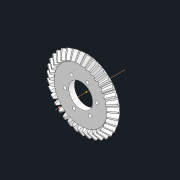
# Autodesk Inventor part: かさ歯車2
Saved by Autodesk Inventor 2021 (Build 250183000, 183)
## iProperties
CustomPartVersion: 1
Created: 2021-07-25
Part Number: かさ歯車2
Material: ABS プラスチック
Document SubType Name: Modeling
Designer: yuto6
Categories: <?xml version="1.0" encoding="UTF-16"?> <MemberInstance><Categories><FamilyTemplate><FamilyTemplateParameter ValueType="xs:double" Id="1" ObjectReferenceKey="da_z" ObjectType="kUserParameterObject"/><FamilyTemplateParameter ValueType="xs:double" Id="2" ObjectReferenceKey="da_b" ObjectType="kUserParameterObject"/><FamilyTemplateParameter ValueType="xs:double" Id="3" ObjectReferenceKey="da_beta" ObjectType="kUserParameterObject"/><FamilyTemplateParameter ValueType="xs:double" Id="4" ObjectReferenceKey="da_dae" ObjectType="kUserParameterObject"/><FamilyTemplateParameter ValueType="xs:double" Id="5" ObjectReferenceKey="da_ve" ObjectType="kUserParameterObject"/><FamilyTemplateParameter ValueType="xs:double" Id="6" ObjectReferenceKey="da_omega" ObjectType="kUserParameterObject"/><FamilyTemplateParameter ValueType="xs:string" Id="7" ObjectReferenceKey="EAIAABAAAAAAHwAAAAAAAIAAAAAAAAAA" ObjectType="83914240" SubObjectId="SurfaceGeometry"/></FamilyTemplate><ParamToTemplateMap><ParamToTemplate CategoryParameter="//CategoryParameter[@InternalName='046C89C9-8512-4d59-83FE-43B91F4F132A']" TemplateParameter="1"/><ParamToTemplate CategoryParameter="//CategoryParameter[@InternalName='2552DF32-E462-4b46-AEBF-C6C7768E72AC']" TemplateParameter="2"/><ParamToTemplate CategoryParameter="//CategoryParameter[@InternalName='C9EE641D-15FC-4fae-A226-E94C4372FDD7']" TemplateParameter="3"/><ParamToTemplate><ParamToTemplate CategoryParameter="//CategoryParameter[@InternalName='00B6519A-459B-49c7-AD84-2E56D39A5744']" ConstantValue="-0.000000"/></ParamToTemplate><ParamToTemplate><ParamToTemplate CategoryParameter="//CategoryParameter[@InternalName='04B31F0E-C7A6-4894-AA32-9629BEFACF47']" ConstantValue="1.000000"/></ParamToTemplate><ParamToTemplate><ParamToTemplate CategoryParameter="//CategoryParameter[@InternalName='43CBEC2E-7847-49e7-A936-2F7889FCB2D9']" ConstantValue="0.200000"/></ParamToTemplate><ParamToTemplate><ParamToTemplate CategoryParameter="//CategoryParameter[@InternalName='B1EFC894-105D-4ebd-86BF-FA20ED196853']" ConstantValue="0.300000"/></ParamToTemplate><ParamToTemplate><ParamToTemplate CategoryParameter="//CategoryParameter[@InternalName='51175063-3D10-4879-93E8-6246FE8B403D']" ConstantValue="2060000000.000000"/></ParamToTemplate><ParamToTemplate><ParamToTemplate CategoryParameter="//CategoryParameter[@InternalName='A3A52E27-4454-46a9-B0BD-C932399B70AF']" ConstantValue="0.300000"/></ParamToTemplate><ParamToTemplate CategoryParameter="//CategoryParameter[@InternalName='2A200944-5A8C-41ca-B96E-8520D2E510F1']" TemplateParameter="4"/><ParamToTemplate><ParamToTemplate CategoryParameter="//CategoryParameter[@InternalName='1A637F62-92C8-44bc-B81F-10802510B579']" ConstantValue="5.719126"/></ParamToTemplate><ParamToTemplate CategoryParameter="//CategoryParameter[@InternalName='B52DD4BE-6863-48fb-BF58-89EF6F9EC65C']" TemplateParameter="5"/><ParamToTemplate><ParamToTemplate CategoryParameter="//CategoryParameter[@InternalName='3956BFF2-84D2-457d-93C2-9B0613DEBA67']" ConstantValue="1.848193"/></ParamToTemplate><ParamToTemplate CategoryParameter="//CategoryParameter[@InternalName='739CFA02-461B-4bf8-8049-181FCAD8B28F']" TemplateParameter="6"/><ParamToTemplate><ParamToTemplate CategoryParameter="//CategoryParameter[@InternalName='A27E999F-E2CE-4481-8A2A-EBF499C4C3C5']" ConstantValue="-0.000000"/></ParamToTemplate><ParamToTemplate><ParamToTemplate CategoryParameter="//CategoryParameter[@InternalName='9E1B4470-B2D3-4ff1-B813-535BB4CDF51A']" ConstantValue="3520000.000000"/></ParamToTemplate><ParamToTemplate><ParamToTemplate CategoryParameter="//CategoryParameter[@InternalName='F8452263-BFF6-458c-9FB1-07C4B99E95CD']" ConstantValue="11400000.000000"/></ParamToTemplate><ParamToTemplate><ParamToTemplate CategoryParameter="//CategoryParameter[@InternalName='3E3BB259-FD49-497f-8171-6EBC954A3479']" ConstantValue="2.000000"/></ParamToTemplate><ParamToTemplate CategoryParameter="//CategoryParameter[@InternalName='27C3BAF2-7550-4e4b-AE2C-0DB134B7D9B7']" TemplateParameter="7"/></ParamToTemplateMap><Category DisplayName="Gear" InternalName="DC85795E-93AB-48d5-8EEE-5A27447B64BD" Mnemonic="Gear"><CategoryParameter DisplayName="z" InternalName="046C89C9-8512-4d59-83FE-43B91F4F132A" Mnemonic="z"/><CategoryParameter DisplayName="b" InternalName="2552DF32-E462-4b46-AEBF-C6C7768E72AC" Mnemonic="b"/><CategoryParameter DisplayName="||b|" InternalName="C9EE641D-15FC-4fae-A226-E94C4372FDD7" Mnemonic="beta"/><CategoryParameter DisplayName="x" InternalName="00B6519A-459B-49c7-AD84-2E56D39A5744" Mnemonic="x"/><CategoryParameter DisplayName="a*" InternalName="04B31F0E-C7A6-4894-AA32-9629BEFACF47" Mnemonic="a"/><CategoryParameter DisplayName="c*" InternalName="43CBEC2E-7847-49e7-A936-2F7889FCB2D9" Mnemonic="c"/><CategoryParameter DisplayName="r|.f|*" InternalName="B1EFC894-105D-4ebd-86BF-FA20ED196853" Mnemonic="rf"/><CategoryParameter DisplayName="E" InternalName="51175063-3D10-4879-93E8-6246FE8B403D" Mnemonic="E"/><CategoryParameter DisplayName="||m|" InternalName="A3A52E27-4454-46a9-B0BD-C932399B70AF" Mnemonic="mi"/><Category DisplayName="BevelGear" InternalName="0C98F69A-0C2B-4791-B2FE-7691BB227E77" Mnemonic="BevelGear"><CategoryParameter DisplayName="d|.ae|" InternalName="2A200944-5A8C-41ca-B96E-8520D2E510F1" Mnemonic="dae"/><CategoryParameter DisplayName="d|.ai|" InternalName="1A637F62-92C8-44bc-B81F-10802510B579" Mnemonic="dai"/><CategoryParameter DisplayName="J|.e|" InternalName="B52DD4BE-6863-48fb-BF58-89EF6F9EC65C" Mnemonic="ve"/><CategoryParameter DisplayName="J|.i|" InternalName="3956BFF2-84D2-457d-93C2-9B0613DEBA67" Mnemonic="vi"/><CategoryParameter DisplayName="||S|" InternalName="739CFA02-461B-4bf8-8049-181FCAD8B28F" Mnemonic="omega"/><CategoryParameter DisplayName="x|.t|" InternalName="A27E999F-E2CE-4481-8A2A-EBF499C4C3C5" Mnemonic="xt"/><CategoryParameter DisplayName="||s||.Flim|" InternalName="9E1B4470-B2D3-4ff1-B813-535BB4CDF51A" Mnemonic="sFlim"/><CategoryParameter DisplayName="||s||.Hlim|" InternalName="F8452263-BFF6-458c-9FB1-07C4B99E95CD" Mnemonic="sHlim"/><CategoryParameter DisplayName="種類" InternalName="3E3BB259-FD49-497f-8171-6EBC954A3479" Mnemonic="type"/><CategoryParameter DisplayName="PitchDiameter" InternalName="27C3BAF2-7550-4e4b-AE2C-0DB134B7D9B7" Mnemonic="IDS_PITCHDIAM"/></Category></Category></Categories></MemberInstance>
Mass: 17.814 g
Surface Area: 98.5592 cm^2
Volume: 16.8057 cm^3
Density: 1.06 g/cm^3
Appearance: 滑らか - 白
Author: yuto6
Autodesk Inventor part; units mm, degrees
ref_plane "メッシュ平面2" through (0, 0, 0) normal (0.9959743, 0.0896393, 0) x (0, 0, 1)
sketch "歯のボディ スケッチ" plane through (0, 0, 0) normal (1, 0, 0) x (0, 1, 0)
  line L0 (0, 0) -> (33.605, -26.953) construction
  line L1 (33.605, -26.953) -> (36.1625, -23.3725)
  line L2 (36.1625, -23.3725) -> (0, 0) construction
  line L3 (35, -25) -> (0, 0) construction
  line L4 (26.5733, -21.3132) -> (28.5956, -18.4819)
  line L5 (33.605, -26.953) -> (26.5733, -21.3132)
  line L6 (36.1625, -23.3725) -> (28.5956, -18.4819)
  line L7 (0, -32.3655) -> (0, 5.3943) projected
  line L8 (0, -25) -> (36.1625, -25) construction
  dimension "d0" = 70
  dimension "d1" = 67.2101
  dimension "d2" = 72.325
  dimension "d3" = 9
  dimension "d4" = 23.3725
  constraints: 16 end point, 4 point on line, 3 perpendicular, 2 collinear, 1 horizontal alignment, 1 vertical alignment
  measures "d0" diameter of L3.start L7
  measures "d1" diameter of L0.end L7
  measures "d2" diameter of L1.end L7
  measures "d3" distance between parallel lines of L1 L4
  measures "d4" vertical distance of L1.end L0.start
revolve "歯のボディ" add sketch "歯のボディ スケッチ" angle 360 about axis through (0, 0, 0) along (0, 0, 1)
ref_plane "歯の平面" through (0, 35, -25) normal (0, -0.8137335, 0.5812382) x (1, 0, 0)
sketch "開始スケッチ" plane through (0, 35, -25) normal (0, -0.8137335, 0.5812382) x (1, 0, 0)
  line L0 (0, -76.4044) -> (0, 16.6276) projected
  arc A0 (-0.6975, -2.928) -> (-3.1799, 3.2404) centre (-21.4439, -7.6935) ccw
  arc A1 (3.1799, 3.2404) -> (0.6975, -2.928) centre (21.4439, -7.6935) ccw
  line L1 (-0.6975, -2.928) -> (0.6975, -2.928)
  arc A2 (3.1799, 3.2404) -> (-3.1799, 3.2404) centre (0, -60.2163) ccw
  dimension "d7" = 21.2867
  dimension "d8" = 21.4439
  dimension "d9" = 52.5228
  dimension "d57" = 63.5363
  dimension "d58" = 57.2883
  constraints: 6 point on circle, 3 centre point, 3 symmetric about line, 2 end point, 1 coincident, 1 perpendicular, 1 other
  measures "d7" radius of A0
  measures "d8" horizontal distance of point (0, -60.216) A0.centre
  measures "d9" vertical distance of point (0, -60.216) A0.centre
  measures "d57" radius of A2
  measures "d58" distance from line of A2.centre L1
ref_plane "終了側平面" through (0, 27.4974, -19.641) normal (0, -0.8137335, 0.5812382) x (1, 0, 0)
sketch "終了側スケッチ" plane through (0, 27.4974, -19.641) normal (0, -0.8137335, 0.5812382) x (1, 0, 0)
  line L0 (0, -60.3318) -> (0, 13.1298) projected
  arc A0 (-0.548, -2.3004) -> (-2.4983, 2.5458) centre (-16.8472, -6.0443) ccw
  arc A1 (2.4983, 2.5458) -> (0.548, -2.3004) centre (16.8472, -6.0443) ccw
  line L1 (-0.548, -2.3004) -> (0.548, -2.3004)
  arc A2 (2.4983, 2.5458) -> (-2.4983, 2.5458) centre (0, -47.3083) ccw
  dimension "d12" = 16.7237
  dimension "d15" = 16.8472
  dimension "d16" = 41.264
  dimension "d59" = 49.9166
  dimension "d60" = 45.0079
  constraints: 6 point on circle, 3 centre point, 3 symmetric about line, 2 end point, 1 coincident, 1 other
  measures "d12" radius of A0
  measures "d15" horizontal distance of A0.centre point (0, -47.308)
  measures "d16" vertical distance of A0.centre point (0, -47.308)
  measures "d59" radius of A2
  measures "d60" distance from line of A2.centre L1
loft "Loft" cut profiles "開始スケッチ", "終了側スケッチ"
pattern_circular "Circular Pattern" count 35 over 360 about axis through (0, 0, 0) along (0, 0, 1) of "Loft"
sketch3d "3D スケッチ(右)"
ref_plane "終了側平面(右)" through (-5.1623, 27.0084, -19.641) normal (0.152769, -0.7992645, 0.5812382) x (0.9822191, 0.1877384, 0)
sketch "終了側スケッチ(右)" plane through (-5.1623, 27.0084, -19.641) normal (0.152769, -0.7992645, 0.5812382) x (0.9822191, 0.1877384, 0)
  arc A0 (-0.548, -2.3004) -> (-2.4983, 2.5458) centre (-16.8472, -6.0443) ccw
  line L0 (0, -65.6359) -> (0, 18.4339) projected
  arc A1 (2.4983, 2.5458) -> (0.548, -2.3004) centre (16.8472, -6.0443) ccw
  line L1 (-0.548, -2.3004) -> (0.548, -2.3004)
  arc A2 (2.4983, 2.5458) -> (-2.4983, 2.5458) centre (0, -47.3083) ccw
  dimension "d70" = 16.8472
  dimension "d71" = 41.264
  dimension "d72" = 16.7237
  dimension "d73" = 45.0079
  dimension "d74" = 49.9166
  constraints: 6 point on circle, 3 centre point, 3 symmetric about line, 2 end point, 1 coincident, 1 perpendicular, 1 other
  measures "d70" horizontal distance of A2.centre A0.centre
  measures "d71" vertical distance of point (0, -47.308) A0.centre
  measures "d72" radius of A0
  measures "d73" distance from line of point (0, -47.308) L1
  measures "d74" radius of A2
feature "ロフト(右)" [suppressed]
pattern_circular "放射状パターン(右)" [suppressed]
sketch3d "3D スケッチ(左)"
ref_plane "終了側平面(左)" through (5.2103, 27.0084, -19.6876) normal (-0.1540308, -0.7984503, 0.5820237) x (0.9818962, -0.1894197, 0)
sketch "終了側スケッチ(左)" plane through (5.2103, 27.0084, -19.6876) normal (-0.1540308, -0.7984503, 0.5820237) x (0.9818962, -0.1894197, 0)
  line L0 (0, -69.242) -> (0, 22.1112) projected
  arc A0 (-0.548, -2.2677) -> (-2.4983, 2.5784) centre (-16.8472, -6.0116) ccw
  arc A1 (2.4983, 2.5784) -> (0.548, -2.2677) centre (16.8472, -6.0116) ccw
  line L1 (-0.548, -2.2677) -> (0.548, -2.2677)
  ellipse E0 centre (0, -15.029) end of major axis (28.5956, -15.029) minor radius 16.6433 projected
  arc A2 (2.4983, 2.5784) -> (-2.4983, 2.5784) centre (0, -47.2756) ccw
  dimension "d56" = 16.6433
  dimension "d30" = 16.7237
  dimension "d31" = 16.8472
  dimension "d32" = 41.264
  dimension "d61" = 49.9166
  dimension "d62" = 45.0079
  constraints: 6 point on circle, 3 centre point, 3 symmetric about line, 2 end point, 1 coincident, 2 other
  measures "d30" radius of A0
  measures "d31" horizontal distance of point (0, -47.276) A0.centre
  measures "d32" vertical distance of A0.centre point (0, -47.276)
  measures "d61" radius of A2
  measures "d62" distance from line of point (0, -47.276) L1
feature "ロフト(左)" [suppressed]
pattern_circular "放射状パターン(左)" [suppressed]
sketch "ボディ スケッチ" plane through (0, 0, 0) normal (1, 0, 0) x (0, 1, 0)
  line L0 (0, -28.079) -> (0, -20.3253) projected
  line L1 (33.605, -26.953) -> (26.5733, -21.3132) projected
  line L2 (26.5733, -21.3132) -> (0, -21.3132)
  line L3 (33.605, -26.953) -> (0, -26.953)
  constraints: 4 end point, 2 perpendicular, 2 point on line
revolve "固定ボディ" add sketch "ボディ スケッチ" angle 360 about axis through (0, 0, 0) along (0, 0, 1)
sketch "Sketch6" plane through (0, 0, 0) normal (1, 0, 0) x (0, 1, 0)
  line L0 (35, -25) -> (0, 0) projected
  line L1 (0, -32.3655) -> (0, 5.3943) projected
surface revolve "ピッチ円直径" sketch "Sketch6" angle 360 about axis through (0, 0, 0) along (0, 0, 1) shown no curves L0
sketch "スケッチ8" plane through (0, 0, -26.953) normal (0, 0, -1) x (-1, 0, 0)
  point P0 (0, 0)
sketch "スケッチ9" plane through (0, 0, -26.953) normal (0, 0, -1) x (-1, 0, 0)
  circle A0 centre (0, 0) radius 22
  dimension "d94" = 44
  constraints: 1 centre point, 1 coincident
  measures "d94" diameter of A0
extrude "押し出し1" add sketch "スケッチ9" along normal blind 3
sketch "スケッチ13" plane through (0, 0, -29.953) normal (0, 0, -1) x (-1, 0, 0)
  circle A0 centre (0, 0) radius 20
  dimension "d127" = 40
  constraints: 1 centre point, 1 coincident
  measures "d127" diameter of A0
extrude "押し出し3" add sketch "スケッチ13" along normal blind 14
sketch "スケッチ11" plane through (0, 0, -21.3132) normal (0, 0, 1) x (1, 0, 0)
  circle A0 centre (0, 0) radius 12
  dimension "d112" = 24
  constraints: 1 centre point, 1 coincident
  measures "d112" diameter of A0
extrude "押し出し2" cut sketch "スケッチ11" against normal through all
sketch "スケッチ12" plane through (0, 0, -21.3132) normal (0, 0, 1) x (0.9959743, 0.0896393, 0)
  circle A0 centre (0, 0) radius 16
  point P0 (-16, 0)
  point P1 (-8, -13.8564)
  point P2 (8, -13.8564)
  point P3 (16, 0)
  point P4 (8, 13.8564)
  point P5 (-8, 13.8564)
  dimension "d115" = 32
  dimension "d118" = 360
  constraints: 1 coincident, 1 horizontal alignment, 9 other
hole "穴2" at (-15.9356, -1.4342, -21.3132) at (-6.7257, -14.5177, -21.3132) at (9.2099, -13.0835, -21.3132) at (15.9356, 1.4342, -21.3132) at (6.7257, 14.5177, -21.3132) at (-9.2099, 13.0835, -21.3132) direction (0, 0, -1) diameter 3.2 end through all clearance for "Socket Head Cap Screw" size "M3" standard "Ansi Metric M Profile"
chamfer "面取り2" distance 1 angle 45 1 edges at (20, 0, -43.953)
sketch "スケッチ14" plane through (0, 0, -43.953) normal (0, 0, -1) x (-1, 0, 0)
  circle A0 centre (0, 0) radius 49.679
  constraints: 1 centre point, 1 coincident
extrude "押し出し4" cut sketch "スケッチ14" against normal up to surface (17 mm away)
equation "\"d0\" = da_de"
equation "\"d1\" = da_dfe"
equation "\"d2\" = da_dae"
equation "\"d3\" = da_b"
equation "\"d4\" = da_ve"
equation "\"d7\" = fd_rr"
equation "\"d8\" = fd_x"
equation "\"d9\" = fd_y"
equation "\"d57\" = 0.5 * fd_dva + 0.3 * da_he"
equation "\"d58\" = 0.5 * fd_dva - 1.12 * da_he"
equation "\"da_teethtype\" = 0"
equation "\"da_b\" = 9"
equation "\"da_de\" = 70"
equation "\"da_dae\" = 72.32495"
equation "\"da_dfe\" = 67.21006"
equation "\"da_le\" = 43.01163"
equation "\"da_omega\" = 90deg"
equation "\"da_beta\" = 0"
equation "\"da_delta\" = 54.462322deg"
equation "\"da_alpha\" = 20deg"
equation "\"da_he\" = 4.4"
equation "\"da_ve\" = 23.37253"
equation "\"da_zv\" = 60.216277"
equation "\"fd_loft\" = da_b + 0.05 * da_he"
equation "\"fd_x\" = fd_x1 + fd_x2"
equation "\"fd_y\" = fd_y1 - fd_y2"
equation "\"fd_dd\" = fd_dva - 0.8 * da_he"
equation "\"da_dvw\" = 120.43255"
equation "\"d11\" = fd_loft"
equation "\"da_dm\" = 62.6764"
equation "\"da_x\" = 0"
equation "\"da_m\" = 2"
equation "\"d50\" = da_omega"
equation "\"fd_rr\" = 21.286682"
equation "\"fd_dva\" = 124.432554"
equation "\"fd_x1\" = 1.588065"
equation "\"fd_x2\" = 19.855864"
equation "\"fd_y1\" = 60.195332"
equation "\"fd_y2\" = 7.672517"
body "Solid1"
body "Srf1"
